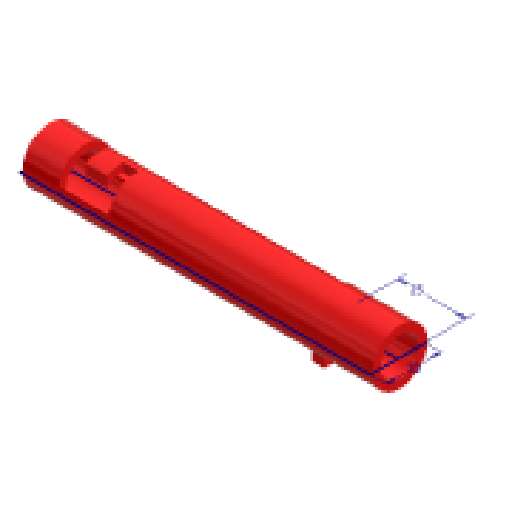
# Autodesk Inventor part: astaoscilla2_306
Saved by Autodesk Inventor 2024 (Build 280153000, 153)
## iProperties
Created: 2024-04-19
Part Number: astaoscilla2_306
Material: Generico
Document SubType Name: Modeling
Designer: Kelly
Density: 1 g/cm^3
Appearance: Liscia - Rosso
Author: Kelly
Autodesk Inventor part; units mm, degrees
ref_plane "YZ Plane" through (0, 0, 0) normal (1, 0, 0) x (0, 1, 0)
ref_plane "XY Plane" through (0, 0, 0) normal (0, 0, 1) x (1, 0, 0)
sketch "Schizzo2" plane through (0, 0, 0) normal (1, 0, 0) x (0, 1, 0)
  circle A0 centre (0, -11) radius 10
  point P0 (0, 0)
  dimension "d4" = 11
  dimension "d5" = 20
  constraints: 1 centre point
  measures "d4" distance of point (0, 0) A0.centre
  measures "d5" diameter of A0
extrude "Estrusione1" add sketch "Schizzo2" against normal blind 128
shell "Svuotamento1" thickness 3 removed faces 2 at (0, -3.2365, -10.2023) at (-128, -3.2365, -10.2023)
sketch "Schizzo1" plane through (0, 0, 0) normal (0, 1, 0) x (-1, 0, 0)
  line L0 (0, 0) -> (0, -20)
  line L1 (0, -10) -> (128, -10)
  line L2 (128, 0) -> (128, -20)
  line L3 (0, -20) -> (25, -20)
  line L4 (25, -20) -> (128, -20)
  line L5 (128, 0) -> (0, 0)
  dimension "d0" = 20
  dimension "d3" = 25
  constraints: 12 end point, 3 horizontal, 2 vertical, 1 midpoint, 1 parallel
  measures "d0" distance of L0.start L0.end
  measures "d3" distance of L0.end L3.end
ref_plane "Piano di lavoro7" through (0, 10, -11) normal (0, 1, 0) x (-1, 0, 0)
sketch "Schizzo13" plane through (0, 10, -11) normal (0, 1, 0) x (-1, 0, 0)
  line L0 (24.8317, -9) -> (114.8317, -9)
  line L1 (24.8317, -9) -> (24.8317, -4)
  line L2 (24.8317, -4) -> (109.8317, -4)
  line L3 (114.8317, -9) -> (114.8317, 9.8878)
  line L4 (0, 7) -> (128, 7) projected
  line L5 (109.8317, -4) -> (109.8317, 4.8878)
  line L6 (114.8317, 9.8878) -> (96.5899, 9.8878)
  line L7 (96.5899, 9.8878) -> (96.5899, -1.1122)
  line L8 (96.5899, -1.1122) -> (102.0899, -1.1122)
  line L9 (102.0899, -1.1122) -> (102.0899, 4.8878)
  line L10 (109.8317, 4.8878) -> (102.0899, 4.8878)
  point P0 (0, 11)
  dimension "d59" = 90
  dimension "d60" = 5
  dimension "d61" = 85
  dimension "d62" = 6
  dimension "d63" = 5
  dimension "d64" = 5.5
  dimension "d65" = 11
  constraints: 20 end point, 6 perpendicular, 1 horizontal, 1 parallel, 1 vertical
  measures "d59" distance of L0.start L0.end
  measures "d60" distance of L0.start L1.end
  measures "d61" distance of L1.end L2.end
  measures "d62" distance of L8.end L9.end
  measures "d63" distance between parallel lines of L10 L6
  measures "d64" distance of L7.end L8.end
  measures "d65" distance between parallel lines of L4 L2
extrude "Estrusione7" cut sketch "Schizzo13" against normal blind 11.25
ref_plane "Piano di lavoro8" through (0, -10, -11) normal (0, 1, 0) x (-1, 0, 0)
sketch "Schizzo14" plane through (0, -10, -11) normal (0, 1, 0) x (-1, 0, 0)
  line L0 (25.2013, -2.0707) -> (29.7013, -2.0707)
  line L1 (29.7013, -2.0707) -> (29.7013, 2.4293)
  line L2 (29.7013, 2.4293) -> (25.2013, 2.4293)
  line L3 (25.2013, 2.4293) -> (25.2013, -2.0707)
  point P0 (0, 11)
  dimension "d68" = 4.5
  dimension "d69" = 4.5
  constraints: 8 end point, 2 parallel, 1 horizontal, 1 perpendicular
  measures "d68" distance of L0.end L1.end
  measures "d69" distance of L0.start L0.end
extrude "Estrusione8" add sketch "Schizzo14" along normal blind 2.5 and the other way blind 5
